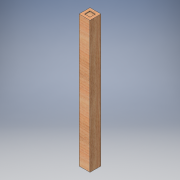
# Autodesk Inventor part: LegStandard
Saved by Autodesk Inventor 2016 (Build 200138000, 138)
## iProperties
Created: 2016-02-09
Part Number: LegStandard
Material: Wood (Birch)
Document SubType Name: Modeling
Designer: ron
Density: 0.55 g/cm^3
Appearance: Birch - Natural Polished
Mass: 864.11 g
Surface Area: 1293.55 cm^2
Volume: 1571.11 cm^3
Author: ron
Autodesk Inventor part; units mm, degrees
ref_plane "YZ Plane" through (0, 0, 0) normal (1, 0, 0) x (0, 1, 0)
ref_plane "XZ Plane" through (0, 0, 0) normal (0, 1, 0) x (-1, 0, 0)
ref_plane "XY Plane" through (0, 0, 0) normal (0, 0, 1) x (1, 0, 0)
sketch "Sketch1" plane through (0, 0, 0) normal (1, 0, 0) x (0, 1, 0)
  line L0 (0, 0) -> (609.6, 0)
  line L1 (609.6, 0) -> (609.6, -50.8)
  line L2 (609.6, -50.8) -> (0, -50.8)
  line L3 (0, -50.8) -> (0, 0)
  dimension "d0" = 609.6
  dimension "d1" = 50.8
  constraints: 8 end point, 2 parallel, 1 horizontal, 1 perpendicular
  measures "d0" distance of L1.end L2.end
  measures "d1" distance of L0.end L1.end
extrude "Extrusion1" add sketch "Sketch1" along normal blind 50.8
sketch "Sketch2" plane through (0, 609.6, 0) normal (0, 1, 0) x (1, 0, 0)
  line L0 (12.7, 38.1) -> (38.1, 38.1)
  line L1 (38.1, 38.1) -> (38.1, 12.7)
  line L2 (38.1, 12.7) -> (12.7, 12.7)
  line L3 (12.7, 12.7) -> (12.7, 38.1)
  line L4 (0, 0) -> (0, 50.8) projected
  line L5 (0, 50.8) -> (50.8, 50.8) projected
  dimension "d4" = 25.4
  dimension "d5" = 25.4
  dimension "d6" = 12.7
  dimension "d7" = 12.7
  constraints: 8 end point, 2 parallel, 1 horizontal, 1 perpendicular
  measures "d4" distance of L1.end L2.end
  measures "d5" distance of L0.end L1.end
  measures "d6" distance between parallel lines of L4 L3
  measures "d7" distance between parallel lines of L5 L0
extrude "Extrusion2" cut sketch "Sketch2" against normal blind 3.175
body "Solid1"
